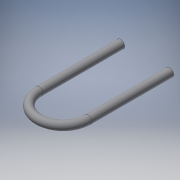
# Autodesk Inventor part: Rope
Saved by Autodesk Inventor 2019 (Build 230136000, 136)
## iProperties
Created: 2020-09-25
Part Number: Rope
Material: Generic
Document SubType Name: Modeling
Designer: nicolas
Density: 1 g/cm^3
Appearance: Default
Author: nicolas
Autodesk Inventor part; units mm, degrees
ref_plane "YZ Plane" through (0, 0, 0) normal (1, 0, 0) x (0, 1, 0)
ref_plane "XZ Plane" through (0, 0, 0) normal (0, 1, 0) x (-1, 0, 0)
ref_plane "XY Plane" through (0, 0, 0) normal (0, 0, 1) x (1, 0, 0)
sketch "Sketch5" plane through (0, 0, 0) normal (0, 0, 1) x (1, 0, 0)
  circle A0 centre (3, 0) radius 0.5
  line L0 (0, -0.7) -> (0, 0.7) projected
  point P0 (0, 0)
  dimension "d8" = 1
  dimension "d9" = 3
  constraints: 1 centre point
  measures "d8" diameter of A0
  measures "d9" distance of point (0, 0) A0.centre
revolve "Revolution1" add sketch "Sketch5" angle 180 about axis through (0, -10, 0) along (0, -1, 0)
sketch "Sketch6" plane through (3, 0, 0) normal (0, 0, -1) x (-1, 0, 0)
  circle A0 centre (0, 0) radius 0.5 projected
  circle A1 centre (6, 0) radius 0.5 projected
  point P0 (3, 0)
extrude "Extrusion1" add sketch "Sketch6" along normal blind 10
body "Solid2"
